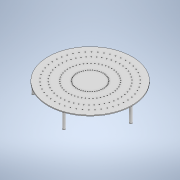
# Autodesk Inventor part: bottom_mesh
Saved by Autodesk Inventor 2020 (Build 240168000, 168)
## iProperties
Created: 2022-08-30
Part Number: bottom_mesh
Material: Generic
Document SubType Name: Modeling
Designer: Intuito_PC
Density: 1 g/cm^3
Appearance: Default
Author: Intuito_PC
Autodesk Inventor part; units mm, degrees
ref_plane "YZ Plane" through (0, 0, 0) normal (1, 0, 0) x (0, 1, 0)
ref_plane "XZ Plane" through (0, 0, 0) normal (0, 1, 0) x (-1, 0, 0)
ref_plane "XY Plane" through (0, 0, 0) normal (0, 0, 1) x (1, 0, 0)
sketch "Sketch1" plane through (0, 0, 0) normal (0, 1, 0) x (-1, 0, 0)
  circle A0 centre (0, 0.4178) radius 250
  line L0 (0, 0.4178) -> (250, 0.4178)
  line L1 (0, 0.4178) -> (77.2542, -237.3464)
  line L2 (0, 0.4178) -> (-202.2542, -146.5286)
  line L3 (0, 0.4178) -> (-202.2542, 147.3641)
  line L4 (0, 0.4178) -> (77.2542, 238.1819)
  circle A1 centre (77.2542, 238.1819) radius 10
  circle A2 centre (250, 0.4178) radius 10
  circle A3 centre (77.2542, -237.3464) radius 10
  circle A4 centre (-202.2542, -146.5286) radius 10
  circle A5 centre (-202.2542, 147.3641) radius 10
  circle A6 centre (250, 0.4178) radius 9
  circle A7 centre (77.2542, -237.3464) radius 9
  circle A8 centre (-202.2542, -146.5286) radius 9
  circle A9 centre (-202.2542, 147.3641) radius 9
  circle A10 centre (77.2542, 238.1819) radius 9
  point P0 (0, 0)
  dimension "d0" = 500
  dimension "d1" = 72
  dimension "d2" = 72
  dimension "d3" = 72
  dimension "d4" = 72
  dimension "d5" = 20
  dimension "d6" = 20
  dimension "d7" = 20
  dimension "d8" = 20
  dimension "d9" = 20
  dimension "d12" = 1
  dimension "d13" = 1
  dimension "d14" = 1
  dimension "d15" = 1
  dimension "d16" = 1
  constraints: 11 centre point, 10 end point, 5 coincident, 5 point on circle, 1 horizontal
  measures "d0" diameter of A0
  measures "d1" angle of L4 L0
  measures "d2" angle of L3 L4
  measures "d3" angle of L1 L0
  measures "d4" angle of L3 L2
  measures "d5" diameter of A1
  measures "d6" diameter of A2
  measures "d7" diameter of A3
  measures "d8" diameter of A4
  measures "d9" diameter of A5
  measures "d12" radial gap between concentric circles of A2 A6
  measures "d13" radial gap between concentric circles of A3 A7
  measures "d14" radial gap between concentric circles of A4 A8
  measures "d15" radial gap between concentric circles of A5 A9
  measures "d16" radial gap between concentric circles of A1 A10
extrude "Extrusion2" add sketch "Sketch1" against normal blind 5 contours L0 A6 A0 | A0 A6 L0 | A6 L0 A2 A0 | A0 A2 L0 A6 | A2 L0 L4 A1 A0 | A0 A3 L1 L0 A2 | A1 L4 A10 A0 | A0 A7 L1 A3 | L1 A3 A0 A4 L2 | L2 A4 A0 A5 L3 | L3 A5 A0 A1 L4 | A10 L4 A0 | A1 A0 A10 L4 | A0 L1 A7 | L1 A7 A0 A3 | A4 A0 A8 L2 | L2 A8 A0 A4 | A5 A0 A9 L3 | L3 A9 A0 A5 | L4 A10 A0 | A0 A7 L1 | A8 A0 L2 | L2 A0 A8 | A9 A0 L3 | L3 A0 A9
sketch "Sketch2" plane through (0, -5, 0.4178) normal (0, -1, 0) x (1, 0, 0)
  circle A0 centre (0, -0.4178) radius 236.9512
  circle A1 centre (242.5298, 0) radius 7.4702
  circle A2 centre (0, 0) radius 250 projected
  line L0 (250, 0) -> (0, 0)
  line L1 (0, 0) -> (-202.2542, -146.9463)
  line L2 (0, 0) -> (77.2542, 237.7641)
  line L3 (0, 0) -> (-202.2542, 146.9463)
  circle A3 centre (75.1664, -231.3384) radius 5.8951
  circle A4 centre (-196.6859, -142.9006) radius 5.9206
  circle A5 centre (-244.3431, 0) radius 7.3923
  circle A6 centre (-196.6859, 142.9006) radius 6.4117
  circle A7 centre (75.1664, 231.3384) radius 6.7565
  circle A8 centre (0, 0) radius 250
  line L4 (76.9881, -236.9449) -> (77.2542, -237.7641)
  dimension "d21" = 72
  dimension "d24" = 72
  dimension "d25" = 72
  constraints: 10 end point, 5 centre point, 5 point on circle, 3 point on line, 2 coincident, 1 concentric, 1 horizontal, 1 horizontal alignment, 1 tangent, 9 other
  measures "d21" angle of L2 L0
  measures "d24" angle of L1 L3
  measures "d25" angle of L3 L2
extrude "Extrusion4" add sketch "Sketch2" along normal blind 90 contours A0 A1 L0 | A0 L0 A1 | L0 A1 A0 | A0 A1 L0 | A3 | A7 L2 A0 | A0 L2 A7 | L2 A0 A7 | A4 L1 A0 | L2 A7 A0 | L1 A4 | A0 A6 L3 | L3 A6 | A5 A2 | A2 A5
sketch "Sketch3" plane through (242.5298, -5, 0.4178) normal (0, -1, 0) x (1, 0, 0)
  point P0 (-242.5298, -0.4178)
  point P1 (-327.9491, -154.2913)
  point P2 (-304.4968, -112.324)
  point P3 (-282.2789, -67.8882)
  point P4 (-345.2297, -185.1495)
hole "Hole1" at (-85.4193, -5, -153.8735) at (-61.967, -5, -111.9063) at (-39.7491, -5, -67.4704) at (-102.6999, -5, -184.7318) direction (0, 1, 0) diameter 5 depth 10 tip angle 118
pattern_circular "Circular Pattern1" count 50 over 360 about axis through (0, 0, 0.4178) along (0, -1, 0) of "Hole1"
body "Solid2"
